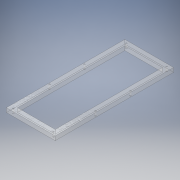
# Autodesk Inventor part: case_top_cover_slot
Saved by Autodesk Inventor 2019 (Build 230136000, 136)
## iProperties
Created: 2019-02-16
Part Number: case_top_cover_slot
Material: Acrylic, Clear
Document SubType Name: Modeling
Designer: suchanek
Density: 1.19 g/cm^3
Appearance: Transparent - Clear
Author: suchanek
Autodesk Inventor part; units mm, degrees
ref_plane "YZ Plane" through (0, 0, 0) normal (1, 0, 0) x (0, 1, 0)
ref_plane "XZ Plane" through (0, 0, 0) normal (0, 1, 0) x (-1, 0, 0)
ref_plane "XY Plane" through (0, 0, 0) normal (0, 0, 1) x (1, 0, 0)
sketch "Sketch1" plane through (0, 0, 0) normal (0, 1, 0) x (-1, 0, 0)
  line L0 (-27, 77) -> (27, 77)
  line L1 (27, 77) -> (27, -77)
  line L2 (27, -77) -> (-27, -77)
  line L3 (-27, -77) -> (-27, 77)
  line L4 (-27, 77) -> (27, -77) construction
  line L5 (27, 77) -> (-27, -77) construction
  line L6 (-35, 85) -> (35, 85)
  line L7 (35, 85) -> (35, -85)
  line L8 (35, -85) -> (-35, -85)
  line L9 (-35, -85) -> (-35, 85)
  line L10 (-35, 85) -> (35, -85) construction
  line L11 (35, 85) -> (-35, -85) construction
  circle A0 centre (28.875, -81.087) radius 0.9
  circle A1 centre (33, -25) radius 0.9
  line L12 (0, 0) -> (0, -26.4871)
  line L13 (0, 0) -> (15.9434, 0)
  circle A2 centre (-28.875, -81.087) radius 0.9
  circle A3 centre (-33, -25) radius 0.9
  circle A4 centre (28.875, 81.087) radius 0.9
  circle A5 centre (33, 25) radius 0.9
  circle A6 centre (-28.875, 81.087) radius 0.9
  circle A7 centre (-33, 25) radius 0.9
  dimension "d0" = 8
  dimension "d1" = 8
  dimension "d2" = 70
  dimension "d3" = 170
  dimension "d6" = 1.8
  dimension "d7" = 1.8
  dimension "d8" = 57.75
  dimension "d9" = 33
  dimension "d10" = 25
  constraints: 28 end point, 8 centre point, 6 symmetric about line, 5 midpoint, 4 parallel, 3 horizontal, 2 perpendicular, 1 vertical, 6 other
  measures "d0" distance between parallel lines of L8 L2
  measures "d1" distance between parallel lines of L7 L1
  measures "d2" distance of L7.end L8.end
  measures "d3" distance of L6.end L7.end
  measures "d6" diameter of A0
  measures "d7" diameter of A1
  measures "d8" distance of A2.centre A0.centre
  measures "d9" distance from line of L12 A1.centre
  measures "d10" distance from line of L13 A1.centre
extrude "Extrusion1" add sketch "Sketch1" along normal blind 6
equation "\"d1\" = d0"
body "Solid1"
